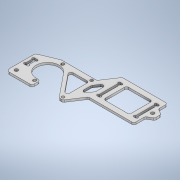
# Autodesk Inventor part: Ankle_side_frame
Saved by Autodesk Inventor 2020.4 (Build 244396000, 396)
## iProperties
Created: 2021-10-01
Part Number: Ankle_side_frame
Material: アルミニウム 2014-T4
Document SubType Name: Modeling
Designer: Masato Kubotera
Density: 2.8 g/cm^3
Appearance: 滑らか - 淡い灰色
Description: A2017 T2
Mass: 9.96642 g
Surface Area: 50.588 cm^2
Volume: 3.55944 cm^3
Author: Masato Kubotera
Autodesk Inventor part; units mm, degrees
ref_plane "YZ Plane" through (0, 0, 0) normal (1, 0, 0) x (0, 1, 0)
ref_plane "XZ Plane" through (0, 0, 0) normal (0, 1, 0) x (-1, 0, 0)
ref_plane "XY Plane" through (0, 0, 0) normal (0, 0, 1) x (1, 0, 0)
sketch "スケッチ1" plane through (0, 0, 0) normal (0, 0, 1) x (1, 0, 0)
  line L0 (28, 13.5) -> (1, 13.5) construction
  line L1 (1, 13.5) -> (1, -13.5) construction
  line L2 (1, -13.5) -> (28, -13.5) construction
  line L3 (28, -13.5) -> (28, 13.5) construction
  line L4 (28, 13.5) -> (1, -13.5) construction
  line L5 (1, 13.5) -> (28, -13.5) construction
  circle A0 centre (0, 0) radius 10.5 construction
  arc A1 (0, 16) -> (-12, 10.583) centre (0, 0) ccw construction
  line L6 (1, 0) -> (28, 0) construction
  line L7 (14.5, 13.5) -> (14.5, -13.5) construction
  circle A2 centre (28, 13.5) radius 1.35
  arc A3 (-0.35, 13) -> (2.35, 13) centre (1, 13) ccw
  line L8 (2.35, 13.5) -> (2.35, 13)
  line L9 (-0.35, 13.5) -> (-0.35, 13)
  arc A4 (2.35, 13.5) -> (-0.35, 13.5) centre (1, 13.5) ccw
  line L10 (-12, 10.583) -> (-12, -10.583) construction
  arc A5 (-12, -10.583) -> (0, -16) centre (0, 0) ccw construction
  circle A6 centre (28, -13.5) radius 1.35
  line L11 (-17.5, 5) -> (-14.5, 5) construction
  line L12 (-14.5, 5) -> (-14.5, -5) construction
  line L13 (-14.5, -5) -> (-17.5, -5) construction
  line L14 (-17.5, -5) -> (-17.5, 5) construction
  line L15 (-17.5, 5) -> (-14.5, -5) construction
  line L16 (-14.5, 5) -> (-17.5, -5) construction
  line L17 (-17.51, 5.01) -> (-14.49, 5.01)
  line L18 (-14.49, 5.01) -> (-14.49, 2.91) construction
  line L19 (-14.49, -5.01) -> (-17.51, -5.01)
  line L20 (-17.51, -5.01) -> (-17.51, -2.91) construction
  line L21 (-17.51, 5.01) -> (-14.49, -5.01) construction
  line L22 (-14.49, 5.01) -> (-17.51, -5.01) construction
  arc A7 (-17.51, 5.01) -> (-17.51, 2.91) centre (-17.51, 3.96) ccw
  line L23 (-17.5, 0) -> (-14.5, 0) construction
  line L24 (-16, 5) -> (-16, -5) construction
  arc A8 (-14.49, 2.91) -> (-14.49, 5.01) centre (-14.49, 3.96) ccw
  arc A9 (-17.51, -2.91) -> (-17.51, -5.01) centre (-17.51, -3.96) ccw
  arc A10 (-14.49, -5.01) -> (-14.49, -2.91) centre (-14.49, -3.96) ccw
  line L25 (-17.51, 2.91) -> (-17.51, 5.01) construction
  line L26 (-17.51, -2.91) -> (-17.51, 2.91)
  line L27 (-14.49, -2.91) -> (-14.49, -5.01) construction
  line L28 (-14.49, 2.91) -> (-14.49, -2.91)
  line L29 (-20.5, 8.739) -> (-20.5, -15.7058)
  line L30 (-3.2261, 16) -> (30.4, 16)
  line L31 (8.7023, 11.1) -> (28, 11.1)
  circle A11 centre (28, 13.5) radius 2.4 construction
  circle A12 centre (28, -13.5) radius 2.4 construction
  line L32 (79.5, 25.4) -> (77.5, 25.4) construction
  line L33 (77.5, 25.4) -> (77.5, 3.6) construction
  line L34 (77.5, 3.6) -> (79.5, 3.6) construction
  line L35 (79.5, 3.6) -> (79.5, 25.4) construction
  line L36 (79.5, 25.4) -> (77.5, 3.6) construction
  line L37 (77.5, 25.4) -> (79.5, 3.6) construction
  line L38 (77.49, 25.41) -> (79.51, 25.41)
  line L39 (79.51, 25.41) -> (79.51, 23.31) construction
  line L40 (79.51, 3.59) -> (77.49, 3.59)
  line L41 (77.49, 3.59) -> (77.49, 5.69) construction
  line L42 (77.49, 25.41) -> (79.51, 3.59) construction
  line L43 (79.51, 25.41) -> (77.49, 3.59) construction
  arc A13 (77.49, 25.41) -> (77.49, 23.31) centre (77.49, 24.36) ccw
  line L44 (78.5, 25.4) -> (78.5, 3.6) construction
  line L45 (77.5, 14.5) -> (79.5, 14.5) construction
  arc A14 (79.51, 23.31) -> (79.51, 25.41) centre (79.51, 24.36) ccw
  arc A15 (77.49, 5.69) -> (77.49, 3.59) centre (77.49, 4.64) ccw
  arc A16 (79.51, 3.59) -> (79.51, 5.69) centre (79.51, 4.64) ccw
  line L46 (77.49, 23.31) -> (77.49, 25.41) construction
  line L47 (79.51, 23.31) -> (79.51, 5.69)
  line L48 (79.51, 5.69) -> (79.51, 3.59) construction
  line L49 (77.49, 5.69) -> (77.49, 23.31)
  circle A17 centre (83.5, 15.5) radius 1.6
  line L50 (83.5, 12.0359) -> (80.5, 13.7679) construction
  line L51 (80.5, 13.7679) -> (80.5, 17.2321) construction
  line L52 (80.5, 17.2321) -> (83.5, 18.9641) construction
  line L53 (83.5, 18.9641) -> (86.5, 17.2321) construction
  line L54 (86.5, 17.2321) -> (86.5, 13.7679) construction
  line L55 (86.5, 13.7679) -> (83.5, 12.0359) construction
  line L56 (40, 30.4) -> (82.75, 30.4)
  line L57 (82.75, 30.4) -> (82.75, 21.7065)
  line L58 (82.75, 21.7065) -> (88.5, 18.3868)
  line L59 (88.5, 18.3868) -> (88.5, 12.6132)
  line L60 (88.5, 12.6132) -> (82.75, 9.2935)
  line L61 (82.75, 9.2935) -> (82.75, -1.4)
  line L62 (82.75, -1.4) -> (40, -1.4)
  line L63 (30.4, -16) -> (40, -1.4)
  line L64 (40, 30.4) -> (40, -1.4) construction
  line L65 (32, 9.3861) -> (32, -4.4659)
  line L66 (32, -4.4659) -> (39, 6.1799)
  line L67 (39, 6.1799) -> (39, 19.8861)
  line L68 (39, 19.8861) -> (32, 9.3861)
  line L69 (-17.5, 10) -> (-14.5, 10) construction
  line L70 (-14.5, -10) -> (-17.5, -10) construction
  line L71 (-17.5, 10) -> (-14.5, -10) construction
  line L72 (-14.5, 10) -> (-17.5, -10) construction
  line L73 (40, 30.4) -> (30.4, 16)
  line L74 (30.4, 16) -> (30.4, -16) construction
  line L75 (43, 25.5) -> (45, 25.5) construction
  line L76 (45, 25.5) -> (45, 3.5) construction
  line L77 (45, 3.5) -> (43, 3.5) construction
  line L78 (43, 3.5) -> (43, 25.5) construction
  line L79 (43, 25.5) -> (45, 3.5) construction
  line L80 (45, 25.5) -> (43, 3.5) construction
  line L81 (42.99, 25.51) -> (45.01, 25.51)
  line L82 (45.01, 25.51) -> (45.01, 23.41)
  line L83 (45.01, 3.49) -> (42.99, 3.49)
  line L84 (42.99, 3.49) -> (42.99, 5.59) construction
  line L85 (42.99, 25.51) -> (45.01, 3.49) construction
  line L86 (45.01, 25.51) -> (42.99, 3.49) construction
  line L87 (44, 25.5) -> (44, 3.5) construction
  line L88 (43, 14.5) -> (45, 14.5) construction
  arc A18 (42.99, 25.51) -> (42.99, 23.41) centre (42.99, 24.46) ccw
  arc A19 (45.01, 23.41) -> (45.01, 25.51) centre (45.01, 24.46) ccw
  arc A20 (42.99, 5.59) -> (42.99, 3.49) centre (42.99, 4.54) ccw
  arc A21 (45.01, 3.49) -> (45.01, 5.59) centre (45.01, 4.54) ccw
  line L89 (45.01, 23.41) -> (45.01, 5.59)
  line L90 (42.99, 5.59) -> (42.99, 25.51)
  line L91 (45.01, 5.59) -> (45.01, 3.49) construction
  line L92 (28, 11.1) -> (28, -7.0627)
  line L93 (49, 25.4) -> (49, 3.6)
  line L94 (49, 3.6) -> (73.5, 3.6)
  line L95 (73.5, 3.6) -> (73.5, 25.4)
  line L96 (73.5, 25.4) -> (49, 25.4)
  arc A22 (8.3509, 6.7694) -> (-10.75, 0) centre (0, 0) ccw
  line L97 (8.3509, 6.7694) -> (26.0579, -15.0743)
  arc A23 (26.0579, -15.0743) -> (28, -16) centre (28, -13.5) ccw
  line L98 (8.7023, 11.1) -> (24.4463, -8.3221)
  line L99 (-20.5, 8.739) -> (-3.2261, 16)
  line L100 (-20.5, -15.7058) -> (-18.8868, -18.5)
  line L101 (-14.2679, -16.5) -> (-17.7321, -16.5) construction
  line L102 (-17.7321, -16.5) -> (-19.4641, -13.5) construction
  line L103 (-19.4641, -13.5) -> (-17.7321, -10.5) construction
  line L104 (-17.7321, -10.5) -> (-14.2679, -10.5)
  line L105 (-14.2679, -10.5) -> (-12.5359, -13.5) construction
  line L106 (-12.5359, -13.5) -> (-14.2679, -16.5) construction
  line L107 (3.75, -18.5) -> (-18.8868, -18.5)
  circle A24 centre (-16, -13.5) radius 1.6
  line L108 (28, -16) -> (30.4, -16)
  line L109 (0, -16) -> (30.4, -16) construction
  arc A25 (24.4463, -8.3221) -> (28, -7.0627) centre (26, -7.0627) ccw
  arc A26 (2.35, -13) -> (-0.35, -13) centre (1, -13) ccw
  line L110 (-0.35, -13.5) -> (-0.35, -13)
  arc A27 (-0.35, -13.5) -> (2.35, -13.5) centre (1, -13.5) ccw
  line L111 (2.35, -13.5) -> (2.35, -13)
  arc A28 (-10.75, 0) -> (0, -10.75) centre (0, 0) ccw
  line L112 (0, -10.75) -> (3.75, -10.75)
  line L113 (3.75, -10.75) -> (3.75, -18.5)
  circle A29 centre (1, -13.5) radius 2.75 construction
  point P0 (14.5, 0)
  point P1 (-16, 0)
  point P2 (-16, 0)
  point P3 (78.5, 14.5)
  point P4 (44, 14.5)
  point P5 (-16, 0)
  dimension "d0" = 27
  dimension "d1" = 27
  dimension "d2" = 21
  dimension "d6" = 2.7
  dimension "d9" = 0.5
  dimension "d10" = 1.35
  dimension "d11" = 1
  dimension "d12" = 16
  dimension "d13" = 12
  dimension "d14" = 3
  dimension "d16" = 2.5
  dimension "d18" = 0.01
  dimension "d28" = 3
  dimension "d29" = 4.8
  dimension "d53" = 4.8
  dimension "d54" = 10
  dimension "d55" = 0.01
  dimension "d56" = 1.05
  dimension "d75" = 1.05
  dimension "d76" = 0.01
  dimension "d77" = 0.01
  dimension "d80" = 3.2
  dimension "d86" = 3.25
  dimension "d87" = 2
  dimension "d88" = 2
  dimension "d89" = 5
  dimension "d90" = 2
  dimension "d91" = 6
  dimension "d92" = 2
  dimension "d93" = 5
  dimension "d95" = 1
  dimension "d96" = 5
  dimension "d97" = 21.8
  dimension "d104" = 5
  dimension "d109" = 5
  dimension "d110" = 5
  dimension "d111" = 2
  dimension "d112" = 22
  dimension "d113" = 1.05
  dimension "d115" = 0.01
  dimension "d116" = 0.01
  dimension "d117" = 32.5
  dimension "d118" = 45
  dimension "d120" = 4
  dimension "d121" = 4
  dimension "d122" = 3
  dimension "d124" = 14.5
  dimension "d125" = 5
  dimension "d126" = 5
  dimension "d127" = 4
  dimension "d128" = 4
  dimension "d135" = 17
  dimension "d136" = 20
  dimension "d141" = 0.25
  dimension "d143" = 3
  dimension "d144" = 6
  dimension "d145" = 2
  dimension "d146" = 2
  dimension "d148" = 0.5
  dimension "d149" = 3.2
  dimension "d151" = 2
  dimension "d153" = 5.5
  constraints: 230 end point, 45 parallel, 44 point on circle, 37 midpoint, 30 centre point, 26 symmetric about line, 22 perpendicular, 15 point on line, 15 tangent, 13 horizontal, 11 coincident, 6 vertical, 3 collinear, 1 concentric, 39 other
  measures "d0" distance of L2.end L1.end
  measures "d1" distance of L1.end L0.end
  measures "d2" diameter of A0
  measures "d6" diameter of A2
  measures "d9" distance of A3.centre L0.end
  measures "d10" radius of A4
  measures "d11" distance of point (0, 0) L6.start
  measures "d12" radius of A1
  measures "d13" distance from line of L10 A0.centre
  measures "d14" distance of L12.end L13.end
  measures "d16" distance between parallel lines of L10 L12
  measures "d18" distance between parallel lines of L17 L11
  measures "d28" distance between parallel lines of L29 L14
  measures "d29" diameter of A11
  measures "d53" diameter of A12
  measures "d54" distance between parallel lines of L13 L11
  measures "d55" distance between parallel lines of L14 L25
  measures "d56" radius of A7
  measures "d75" radius of A13
  measures "d76" distance between parallel lines of L32 L38
  measures "d77" distance between parallel lines of L41 L33
  measures "d80" diameter of A17
  measures "d86" distance between parallel lines of L57 L35
  measures "d87" distance between parallel lines of L59 L54
  measures "d88" distance between parallel lines of L58 L53
  measures "d89" horizontal distance of point (83.5, 15.5) point (78.5, 14.5)
  measures "d90" distance between parallel lines of L60 L55
  measures "d91" distance between parallel lines of L55 L52
  measures "d92" distance between parallel lines of L33 L35
  measures "d93" distance between parallel lines of L56 L32
  measures "d95" vertical distance of point (78.5, 14.5) A17.centre
  measures "d96" distance between parallel lines of L62 L34
  measures "d97" distance between parallel lines of L34 L32
  measures "d104" distance between parallel lines of L63 L66
  measures "d109" distance between parallel lines of L11 L69
  measures "d110" distance between parallel lines of L73 L68
  measures "d111" distance of L76.end L77.end
  measures "d112" distance of L75.end L76.end
  measures "d113" radius of A18
  measures "d115" distance between parallel lines of L81 L75
  measures "d116" distance between parallel lines of L84 L78
  measures "d117" distance between parallel lines of L33 L76
  measures "d118" distance from line of L76 point (0, 0)
  measures "d120" distance between parallel lines of L92 L65
  measures "d121" distance between parallel lines of L78 L67
  measures "d122" distance between parallel lines of L64 L78
  measures "d124" distance between parallel lines of L6 L88
  measures "d125" distance between parallel lines of L96 L56
  measures "d126" distance between parallel lines of L62 L94
  measures "d127" distance between parallel lines of L76 L93
  measures "d128" distance between parallel lines of L95 L33
  measures "d135" distance from line of point (-16, 0) L1
  measures "d136" distance between parallel lines of L70 L69
  measures "d141" radial gap between concentric circles of A22 A0
  measures "d143" distance between parallel lines of L97 L98
  measures "d144" distance between parallel lines of L101 L104
  measures "d145" distance between parallel lines of L100 L102
  measures "d146" distance between parallel lines of L107 L101
  measures "d148" distance between parallel lines of L104 L70
  measures "d149" diameter of A24
  measures "d151" radius of A25
  measures "d153" diameter of A29
extrude "押し出し1" add sketch "スケッチ1" along normal blind 2
fillet "フィレット1" radius 2 16 edges at (-20.5, 8.739, 1) (-20.5, -15.7058, 1) (-18.8868, -18.5, 1) (30.4, 16, 1) (40, 30.4, 1) (82.75, 30.4, 1) (82.75, 21.7065, 1) (88.5, 18.3868, 1) (88.5, 12.6132, 1) (82.75, 9.2935, 1) (82.75, -1.4, 1) (40, -1.4, 1) (30.4, -16, 1) (-3.2261, 16, 1) (3.75, -18.5, 1) (3.75, -10.75, 1)
fillet "フィレット2" radius 2 10 edges at (32, 9.3861, 1) (32, -4.4659, 1) (39, 6.1799, 1) (39, 19.8861, 1) (28, 11.1, 1) (49, 25.4, 1) (49, 3.6, 1) (73.5, 3.6, 1) (73.5, 25.4, 1) (8.7023, 11.1, 1)
equation "\"d10\" = 0.5 * d6"
